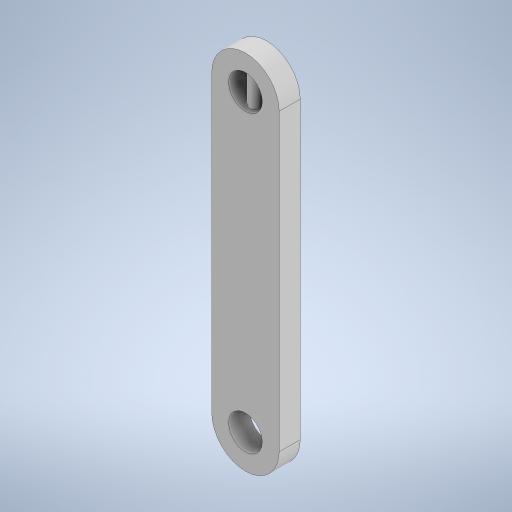
# Autodesk Inventor part: 1-15
Saved by Autodesk Inventor 2024.2 (Build 282272000, 272)
## iProperties
Created: 2024-10-10
Part Number: 1-15
Material: Generic
Document SubType Name: Modeling
Designer: Precisión-04
Density: 1 g/cm^3
Appearance: Default
Author: Precisión-04
Autodesk Inventor part; units mm, degrees
ref_plane "YZ Plane" through (0, 0, 0) normal (1, 0, 0) x (0, 1, 0)
ref_plane "XZ Plane" through (0, 0, 0) normal (0, 1, 0) x (-1, 0, 0)
ref_plane "XY Plane" through (0, 0, 0) normal (0, 0, 1) x (1, 0, 0)
sketch "Sketch1" plane through (0, 0, 0) normal (0, 0, 1) x (1, 0, 0)
  arc A0 (4, 0) -> (-4, 0) centre (0, 0) ccw
  arc A1 (-4, -35) -> (4, -35) centre (0, -35) ccw
  line L0 (0, 0) -> (0, -41.3039) construction
  line L1 (-4, 0) -> (-4, -35)
  line L2 (4, 0) -> (4, -35)
  circle A2 centre (0, 0) radius 2
  circle A3 centre (0, -35) radius 2
  dimension "d0" = 8
  dimension "d1" = 8
  dimension "d2" = 35
  dimension "d3" = 4
  dimension "d4" = 4
  constraints: 6 end point, 4 centre point, 4 point on circle, 3 coincident, 3 vertical, 2 tangent, 1 point on line
  measures "d0" diameter of A0
  measures "d1" diameter of A1
  measures "d2" distance of A1.centre point (0, 0)
  measures "d3" diameter of A2
  measures "d4" diameter of A3
extrude "Extrusion1" add sketch "Sketch1" along normal blind 2.5
sketch "Sketch2" plane through (0, 0, 0) normal (1, 0, 0) x (0, 1, 0)
  line L0 (2, 2.5) -> (2, 0) projected
  line L1 (2, 1.25) -> (-2, 1.25)
  line L2 (-2, 2.5) -> (-2, 0) projected
  line L3 (2, 1.25) -> (-2, 1.25)
  line L4 (-2, 1.25) -> (-2, 2)
  line L5 (-2, 2) -> (2, 2)
  line L6 (2, 2) -> (2, 1.25)
  point P0 (0, 0)
  point P1 (2, 2)
  dimension "d7" = 1.5
  constraints: 10 end point, 2 midpoint, 2 parallel, 1 horizontal, 1 perpendicular, 1 point on line
  measures "d7" diameter of L5 L1
revolve "Revolution1" add sketch "Sketch2" angle 360 about axis through (0, 2, 1.25) along (0, -1, 0)
body "Solid1"
